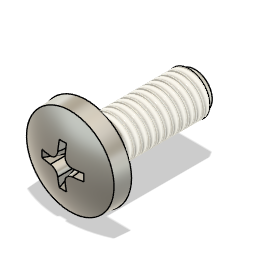
34fcb12c-a30f-4a6b-ad9a-0eb1a66a04d2 (Autodesk Fusion 360 design; units mm, degrees)
description: Parafuso Philips de máquina de cabeça abaulada Tipo I ANSI B18.6.3 3-56 UNF x 0.25
part number: CRBHMSTI ANSI B18.6.3 - 3-56 x 1/4 Aço grau 2 Liso
Autodesk Fusion 360 part; units mm, degrees
sketch "Sketch1" plane through (0, 0, 0) normal (0, 1, 0) x (1, 0, 0)
  line L0 (-1.2573, 0) -> (-1.2573, 6.35)
  line L1 (-1.2573, 6.35) -> (0, 6.35)
  line L2 (0, 6.35) -> (0, -1.4986)
  line L3 (-1.2573, 0) -> (-2.6416, 0)
  line L4 (-2.6416, 0) -> (-2.5594, -0.9398)
  arc A0 (-2.5594, -0.9398) -> (0, -1.4986) centre (0, 4.6419) ccw
  dimension "d9" = 2.5146
  dimension "d66" = 5.2832
  dimension "d106" = 5
  dimension "d113" = 0.9398
  dimension "d119" = 1.4986
  dimension "d120" = 6.35
  constraint perpendicular L0 L1
  constraint collinear origin L2.end L1.end
  constraint perpendicular L0 L3
  constraint coincident origin L3
  constraint vertical L0
  constraint vertical L2
  constraint coincident L2 A0.centre
  measures "d106" angle of L2 L4
  measures "d113" distance of L3 L4.end
  measures "d119" distance of L2.end L3
  measures "d120" distance of origin L1
revolve "Revolve1" add sketch "Sketch1" angle 360 about axis through (0, 0, -6.35) along (0, 0, 1) makes body 1
ref_plane "WorkPlane1" through (0, 0, 1.4986) normal (0, 0, 1) x (1, 0, 0)
sketch "Sketch2" plane through (0, 0, 1.4986) normal (0, 0, 1) x (1, 0, 0)
  line L0 (-0.2159, 0.2159) -> (-1.3081, 0.2159)
  line L1 (-0.2159, -0.2159) -> (-1.3081, -0.2159)
  line L2 (-1.3081, 0.2159) -> (-1.3081, -0.2159)
  line L3 (-0.2159, -0.2159) -> (-0.2159, -1.3081)
  line L4 (-0.2159, -1.3081) -> (0.2159, -1.3081)
  line L5 (0.2159, -0.2159) -> (0.2159, -1.3081)
  line L6 (0.2159, -0.2159) -> (1.3081, -0.2159)
  line L7 (1.3081, -0.2159) -> (1.3081, 0.2159)
  line L8 (0.2159, 0.2159) -> (1.3081, 0.2159)
  line L9 (0.2159, 0.2159) -> (0.2159, 1.3081)
  line L10 (0.2159, 1.3081) -> (-0.2159, 1.3081)
  line L11 (-0.2159, 0.2159) -> (-0.2159, 1.3081)
  dimension "d109" = 360
  dimension "d114" = 0.4318
  dimension "d115" = 2.6162
  constraint vertical L0.start L1.start
  constraint horizontal L0
  constraint horizontal L1
  constraint coincident L0.start L11.start
  constraint vertical L2
  measures "d114" distance of L0 L1
  measures "d115" distance of L2 L7
extrude "Extrude1" add sketch "Sketch2" against normal blind 1.4986 draft -4 separate body makes body 2
draft "Draft1" angle -30 neutral plane through (0, 0, 1.4986) pull (0, 0, 1) 4 faces at (-1.2732, 0.037, 0.9991) (-0.037, -1.2732, 0.9991) (1.2732, -0.037, 0.9991) (0.037, 1.2732, 0.9991) on bodies 2
fillet "Fillet3" radius 0.4318 4 edges at (-0.1635, 0.1635, 0.7493) (0.1635, 0.1635, 0.7493) (0.1635, -0.1635, 0.7493) (-0.1635, -0.1635, 0.7493) on bodies 2
combine "Combine1" operation cut target body 1 tool bodies 2
thread "Thread3" "ANSI Unified Screw Threads 0.099(#3) 3-56 UNF 3-56 UNF 2A" major diameter 2.446 minor diameter 1.9583 pitch 0.4536 angle 60 resizes the face on face at (-1.2511, 0.1252, -2.1167) from (0, 0, -1.1339) to (0, 0, -6.35) on bodies 1
sketch "Sketch5" plane through (0, 0, 0) normal (0, 1, 0) x (1, 0, 0)
  line L0 (0, -1.75) -> (0, -22.5)
  line L1 (0, 6.35) -> (0, -1.4986)
  line L2 (0, 6.35) -> (-1.2824, 6.35)
  line L3 (-1.2824, 6.35) -> (-1.2824, 5.8964)
  line L4 (-1.2824, 5.8964) -> (-1.0122, 6.35)
  dimension "d116" = 1.2824
  dimension "d117" = 0.4536
  dimension "d118" = 0.2703
  constraint coincident L1.start L2.start
  constraint perpendicular L1 L2
  constraint perpendicular L2 L3
  constraint coincident L2 L4.end
  measures "d116" distance of L1.start L3
  measures "d117" distance of L2 L3.end
  measures "d118" distance of L3 L4.end
revolve "Revolve2" cut sketch "Sketch5" angle 360 about axis through (0, 0, -6.35) along (0, 0, 1) bodies 1
equation "d9 = adsk_nomdia"
equation "d31 = -adsk_phildepth"
equation "d66 = adsk_headdia"
equation "d71 = adsk_headh"
equation "adsk_nomlen = 0.25 in"
equation "adsk_headh = 0.059 in"
equation "adsk_headdia = 0.208 in"
equation "adsk_nomdia = 0.099 in"
equation "adsk_phildia = 0.103 in"
equation "adsk_philwidth = 0.017 in"
equation "adsk_phildepth = 0.059 in"
equation "adsk_thrlen = 0.20536 in"
equation "adsk_startlen = 0.0178571 in"
equation "adsk_endpointdia = 0.0797 in"
equation "adsk_ovalh = 0.022 in"
equation "adsk_headang = 5.00 deg"
equation "d106 = max(0.001 deg; adsk_headang)"
equation "d112 = adsk_philwidth"
equation "d113 = adsk_headh - adsk_ovalh"
equation "d114 = adsk_philwidth"
equation "d115 = adsk_phildia"
equation "d116 = adsk_nomdia * 0.51"
equation "d117 = adsk_startlen"
equation "d118 = ( adsk_nomdia * 0.51 ) - ( adsk_endpointdia / 2 )"
equation "d119 = adsk_headh"
equation "d120 = adsk_nomlen"
equation "d122 = min(adsk_thrlen; adsk_nomlen - 0.001 in)"
